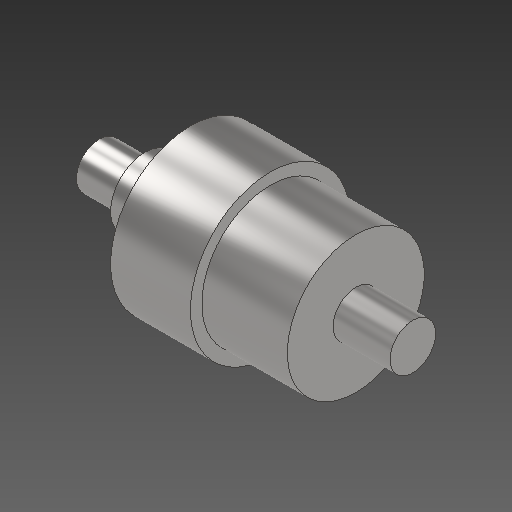
# Autodesk Inventor part: Shaft
Saved by Autodesk Inventor 2021 (Build 250183000, 183)
## iProperties
CustomPartVersion: 1
Created: 2021-03-11
Part Number: Shaft
Material: Steel, Alloy
Document SubType Name: Modeling
Designer: M3rob
Density: 7.73 g/cm^3
Appearance: Semi-Polished
Mass: 4259.33 g
Surface Area: 438.302 cm^2
Volume: 551.013 cm^3
Length: 6.875 in
Author: M3rob
Autodesk Inventor part; units mm, degrees
ref_plane "Start Plane" through (0, 0, 0) normal (1, 0, 0) x (0, 1, 0)
ref_plane "XZ Plane" through (0, 0, 0) normal (0, 1, 0) x (-1, 0, 0)
ref_plane "XY Plane" through (0, 0, 0) normal (0, 0, 1) x (1, 0, 0)
sketch "Main Sketch" plane through (0, 0, 0) normal (0, 0, 1) x (1, 0, 0)
  line L0 (0, 0) -> (174.625, 0)
  line L1 (0, 0) -> (0, 12.7)
  line L2 (25.4, 12.7) -> (25.4, 19.05)
  line L3 (0, 12.7) -> (25.4, 12.7)
  line L4 (50.8, 19.05) -> (50.8, 44.45)
  line L5 (25.4, 19.05) -> (50.8, 19.05)
  line L6 (174.625, 12.7) -> (174.625, 0)
  line L7 (142.875, 12.7) -> (174.625, 12.7)
  line L8 (95.25, 44.45) -> (95.25, 38.1)
  line L9 (50.8, 44.45) -> (95.25, 44.45)
  line L10 (142.875, 38.1) -> (142.875, 12.7)
  line L11 (95.25, 38.1) -> (142.875, 38.1)
  dimension "d3" = 25.4
  dimension "d5" = 38.1
  dimension "d6" = 25.4
  dimension "d7" = 88.9
  dimension "d8" = 76.2
  constraints: 24 end point, 6 vertical, 1 horizontal
  measures "d3" diameter of L3 L0
  measures "d5" diameter of L5 L0
  measures "d6" diameter of L7 L0
  measures "d7" diameter of L9 L0
  measures "d8" diameter of L11 L0
revolve "Revolution1" add sketch "Main Sketch" angle 360 about axis through (0, 0, 0) along (1, 0, 0)
equation "\"Length\" = 174.625"
body "Solid1"
